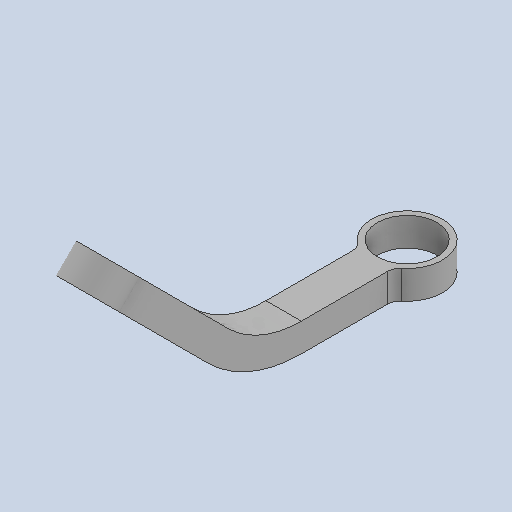
# Autodesk Inventor part: proximal_link_1
Saved by Autodesk Inventor 2024 (Build 280153000, 153)
## iProperties
Created: 2023-10-30
Part Number: proximal_link_1
Material: Generic
Document SubType Name: Modeling
Designer: MATEO
Density: 1 g/cm^3
Appearance: Default
Mass: 23.3464 g
Surface Area: 98.2642 cm^2
Volume: 23.3464 cm^3
Author: MATEO
Autodesk Inventor part; units mm, degrees
ref_plane "YZ Plane" through (0, 0, 0) normal (1, 0, 0) x (0, 1, 0)
sketch "Sketch1" plane through (0, 0, 0) normal (0, 1, 0) x (-1, 0, 0)
  arc A0 (-9.375, 11.7094) -> (9.375, 11.7094) centre (0, 0) ccw
  line L0 (-7.5, 15.6125) -> (-7.5, 22.9904)
  line L1 (7.5, 22.9904) -> (7.5, 15.6125)
  line L2 (7.5, 22.9904) -> (-7.5, 22.9904)
  arc A1 (7.5, 15.6125) -> (9.375, 11.7094) centre (12.5, 15.6125) ccw
  arc A2 (-9.375, 11.7094) -> (-7.5, 15.6125) centre (-12.5, 15.6125) ccw
  point P0 (7.5, 12.9904)
  point P1 (-7.5, 12.9904)
  point P2 (0, 12.9904)
  point P3 (0, 22.9904)
  dimension "d0" = 30
  dimension "d109" = 5
  dimension "d129" = 15
  dimension "d131" = 10
  dimension "d132" = 12.9904
  constraints: 8 point on circle, 6 end point, 5 horizontal alignment, 4 tangent, 3 centre point, 2 point on line, 2 vertical alignment, 1 coincident, 1 equal radius, 1 midpoint, 1 parallel
  measures "d0" diameter of A0
  measures "d109" radius of A1
  measures "d129" distance of L1.start L0.end
  measures "d131" distance from line of L2 point (0, 12.99)
  measures "d132" distance of point (0, 12.99) point (0, 0)
extrude "Extrusion1" add sketch "Sketch1" against normal blind 12
sketch "Sketch22" plane through (-7.5, 0, 22.9904) normal (0, 0, 1) x (1, 0, 0)
  line L0 (0, 0) -> (0, -12) projected
  line L1 (15, -12) -> (0, -12) projected
  line L2 (0, 0) -> (15, 0)
  line L3 (15, 0) -> (15, -12)
  line L4 (15, -12) -> (0, -12)
  line L5 (0, -12) -> (0, 0)
  point P0 (7.5, 0)
  constraints: 8 end point, 2 parallel, 1 horizontal, 1 perpendicular
sketch "Sketch23" plane through (0, 0, 0) normal (1, 0, 0) x (0, 1, 0)
  line L0 (0, 22.9904) -> (-12, 22.9904) projected
  line L1 (-6, 22.9904) -> (-6, 52.2797)
  line L2 (8.6447, 87.635) -> (43.4975, 122.4879)
  arc A0 (8.6447, 87.635) -> (-6, 52.2797) centre (44, 52.2797) ccw
  point P0 (0, 0)
  point P1 (-6, 72.9904)
  dimension "d110" = 50
  dimension "d111" = 70
  dimension "d112" = 135
  dimension "d113" = 50
  constraints: 4 end point, 2 point on circle, 2 point on line, 2 tangent, 1 centre point, 1 midpoint, 1 vertical
  measures "d110" distance of L1.start point (-6, 72.99)
  measures "d111" distance of point (-6, 72.99) L2.end
  measures "d112" angle of L1 L2
  measures "d113" radius of A0
sweep "Sweep2" add profiles "Sketch22" path "Sketch23" path curves L1 A0 L2
ref_plane "Work Plane11" through (7.5, 8.6447, 87.635) normal (0, 0.7071, -0.7071) x (-1, 0, 0)
sketch "Sketch24" plane through (7.5, 8.6447, 87.635) normal (0, 0.7071, -0.7071) x (-1, 0, 0)
  line L0 (0, 49.2893) -> (15, 49.2893) projected
  line L1 (0, 49.2893) -> (15, 49.2893)
  line L2 (0, 49.2893) -> (0, 53.2426)
  line L3 (15, 49.2893) -> (15, 53.2426)
  arc A0 (15, 53.2426) -> (0, 53.2426) centre (7.5, 61.2893) ccw
  point P0 (7.5, -68.08)
  point P1 (7.5, 49.2893)
  point P2 (7.5, 49.2893)
  dimension "d136" = 22
  dimension "d137" = 12
  constraints: 6 end point, 2 midpoint, 2 point on circle, 2 vertical, 1 centre point, 1 collinear, 1 vertical alignment
  measures "d136" diameter of A0
  measures "d137" distance from line of L0 A0.centre
extrude "Extrusion17" add sketch "Sketch24" along normal mid plane 12
sketch "Sketch25" plane through (-7.5, 4.402, 91.8777) normal (0, -0.7071, 0.7071) x (1, 0, 0)
  circle A0 centre (7.5, 61.2893) radius 2.5
  arc A1 (15, 53.2426) -> (0, 53.2426) centre (7.5, 61.2893) ccw projected
  point P0 (7.5, -68.08)
  dimension "d123" = 5
  constraints: 2 coincident, 1 centre point
  measures "d123" diameter of A0
extrude "Extrusion18" cut sketch "Sketch25" along normal through all both and the other way through all
sketch "Sketch26" plane through (0, -12, 0) normal (0, -1, 0) x (1, 0, 0)
  circle A0 centre (0, 0) radius 12.6
  dimension "d133" = 25.2
  constraints: 1 centre point, 1 coincident
  measures "d133" diameter of A0
extrude "Extrusion19" cut sketch "Sketch26" against normal through all
sketch "Sketch28" plane through (7.5, 12.8873, 83.3924) normal (0, 0.7071, -0.7071) x (-1, 0, 0)
  circle A0 centre (7.5, 61.2893) radius 2.5 projected
  circle A1 centre (7.5, 61.2893) radius 8.1
  point P0 (7.5, -68.08)
  dimension "d141" = 16.2
  constraints: 1 centre point, 1 coincident
  measures "d141" diameter of A1
extrude "Extrusion21" cut sketch "Sketch28" against normal blind 5
mirror "Mirror3" about plane through (7.5, 8.6447, 87.635) normal (0, 0.7071, -0.7071) of "Extrusion21"
ref_plane "Work Plane13" through (0, 0, 12.5) normal (0, 0, 1) x (1, 0, 0)
body "Solid1"
